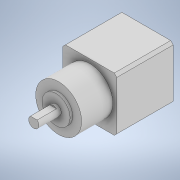
# Autodesk Inventor part: Gearmotor
Saved by Autodesk Inventor 2021 (Build 250183000, 183)
## iProperties
Created: 2024-01-31
Part Number: Gearmotor
Material: Generic
Document SubType Name: Modeling
Designer: Lukas
Density: 1 g/cm^3
Appearance: Default
Author: Lukas
Autodesk Inventor part; units mm, degrees
ref_plane "YZ Plane" through (0, 0, 0) normal (1, 0, 0) x (0, 1, 0)
ref_plane "XZ Plane" through (0, 0, 0) normal (0, 1, 0) x (-1, 0, 0)
ref_plane "XY Plane" through (0, 0, 0) normal (0, 0, 1) x (1, 0, 0)
sketch "Sketch1" plane through (0, 0, 0) normal (0, 0, 1) x (1, 0, 0)
  line L0 (-19.15, 21.15) -> (19.15, 21.15)
  line L1 (21.15, 19.15) -> (21.15, -19.15)
  line L2 (19.15, -21.15) -> (-19.15, -21.15)
  line L3 (-21.15, -19.15) -> (-21.15, 19.15)
  line L4 (-19.15, 21.15) -> (-21.15, 19.15)
  line L5 (-19.15, -21.15) -> (-21.15, -19.15)
  line L6 (21.15, -19.15) -> (19.15, -21.15)
  line L7 (19.15, 21.15) -> (21.15, 19.15)
  point P0 (0, 0)
  point P1 (-21.15, 21.15)
  point P2 (21.15, -21.15)
  point P3 (21.15, 21.15)
  point P4 (-21.15, -21.15)
  point P5 (-21.15, 0)
  point P6 (0, 21.15)
  dimension "d0" = 2
  dimension "d1" = 2
  dimension "d2" = 2
  dimension "d3" = 2
  dimension "d4" = 2
  dimension "d5" = 2
  dimension "d6" = 2
  dimension "d7" = 2
  dimension "d8" = 42.3
  dimension "d9" = 42.3
  constraints: 16 end point, 8 point on line, 2 midpoint, 2 parallel, 1 horizontal, 1 horizontal alignment, 1 perpendicular, 1 vertical alignment
  measures "d0" distance of L0.start point (-21.15, 21.15)
  measures "d1" distance of L3.end point (-21.15, 21.15)
  measures "d2" distance of L2.end point (-21.15, -21.15)
  measures "d3" distance of L3.start point (-21.15, -21.15)
  measures "d4" distance of L1.end point (21.15, -21.15)
  measures "d5" distance of L2.start point (21.15, -21.15)
  measures "d6" distance of L0.end point (21.15, 21.15)
  measures "d7" distance of L1.start point (21.15, 21.15)
  measures "d8" distance between parallel lines of L1 L3
  measures "d9" distance between parallel lines of L0 L2
extrude "Extrusion1" add sketch "Sketch1" along normal blind 44.2
sketch "Sketch2" plane through (0, 0, 44.2) normal (0, 0, 1) x (1, 0, 0)
  circle A0 centre (0, 0) radius 18
  dimension "d12" = 36
  constraints: 1 centre point, 1 coincident
  measures "d12" diameter of A0
extrude "Extrusion2" add sketch "Sketch2" along normal blind 24.5
sketch "Sketch3" plane through (0, 0, 68.7) normal (0, 0, 1) x (1, 0, 0)
  circle A0 centre (0, 0) radius 11
  dimension "d15" = 22
  constraints: 1 centre point, 1 coincident
  measures "d15" diameter of A0
extrude "Extrusion3" add sketch "Sketch3" along normal blind 2
sketch "Sketch4" plane through (0, 0, 70.7) normal (0, 0, 1) x (1, 0, 0)
  circle A0 centre (0, 0) radius 4
  line L0 (-2.6458, 3) -> (2.6458, 3)
  dimension "d18" = 8
  dimension "d19" = 7
  constraints: 2 end point, 2 point on circle, 1 centre point, 1 coincident, 1 horizontal
  measures "d18" diameter of A0
extrude "Extrusion4" add sketch "Sketch4" along normal blind 17.5 contours A0 L0 picked at (-1.0918, 0.7386)
extrude "Extrusion5" add sketch "Sketch4" along normal blind 2.3 contours L0 A0 picked at (-0.6179, 3.1815)
equation "\"d1\" = d0"
equation "\"d2\" = d0"
equation "\"d3\" = d2"
equation "\"d4\" = d0"
equation "\"d5\" = d4"
equation "\"d6\" = d0"
equation "\"d7\" = d6"
equation "\"d9\" = d8"
body "Solid1"
